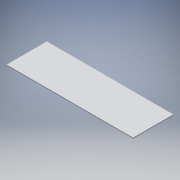
# Autodesk Inventor part: CatapultBase
Saved by Autodesk Inventor 2016 SP1 (Build 200210100, 210)
## iProperties
Created: 2016-01-12
Part Number: CatapultBase
Material: Aluminum 6061
Document SubType Name: Modeling
Designer: steele
Density: 2.7 g/cm^3
Appearance: Aluminum - Flat
Author: steele
Autodesk Inventor part; units mm, degrees
ref_plane "YZ Plane" through (0, 0, 0) normal (1, 0, 0) x (0, 1, 0)
ref_plane "XZ Plane" through (0, 0, 0) normal (0, 1, 0) x (-1, 0, 0)
ref_plane "XY Plane" through (0, 0, 0) normal (0, 0, 1) x (1, 0, 0)
sketch "Sketch1" plane through (0, 0, 0) normal (0, 1, 0) x (-1, 0, 0)
  line L0 (508, 161.5534) -> (-508, 161.5534)
  line L1 (-508, 161.5534) -> (-508, -161.5534)
  line L2 (-508, -161.5534) -> (508, -161.5534)
  line L3 (508, -161.5534) -> (508, 161.5534)
  line L4 (508, 161.5534) -> (-508, -161.5534) construction
  line L5 (-508, 161.5534) -> (508, -161.5534) construction
  point P0 (0, 0)
  dimension "d0" = 1016
  dimension "d1" = 323.1067
  constraints: 12 end point, 2 midpoint, 2 parallel, 1 horizontal, 1 perpendicular
  measures "d0" distance of L0.start L0.end
  measures "d1" distance of L2.end L0.start
extrude "Extrusion1" add sketch "Sketch1" against normal blind 6.35
equation "\"d0\" = catapultBaseWidth"
equation "\"d2\" = catapultBaseDepth"
equation "\"catapultBaseWidth\" = 1016"
equation "\"catapultBaseLength\" = 635"
equation "\"catapultBaseDepth\" = 6.35"
body "Solid1"
